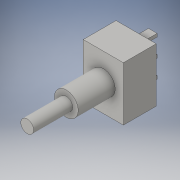
# Autodesk Inventor part: Mini toggle switch
Saved by Autodesk Inventor 2016 (Build 200138000, 138)
## iProperties
Created: 2017-09-11
Part Number: Mini toggle switch
Material: Generic
Document SubType Name: Modeling
Designer: student
Density: 1 g/cm^3
Appearance: Default
Author: student
Autodesk Inventor part; units mm, degrees
ref_plane "YZ Plane" through (0, 0, 0) normal (1, 0, 0) x (0, 1, 0)
ref_plane "XZ Plane" through (0, 0, 0) normal (0, 1, 0) x (-1, 0, 0)
ref_plane "XY Plane" through (0, 0, 0) normal (0, 0, 1) x (1, 0, 0)
sketch "Sketch1" plane through (0, 0, 0) normal (0, 0, 1) x (1, 0, 0)
  line L0 (-4.8133, 6.477) -> (4.8133, 6.477)
  line L1 (4.8133, 6.477) -> (4.8133, -6.477)
  line L2 (4.8133, -6.477) -> (-4.8133, -6.477)
  line L3 (-4.8133, -6.477) -> (-4.8133, 6.477)
  line L4 (-4.8133, 6.477) -> (4.8133, -6.477) construction
  line L5 (4.8133, 6.477) -> (-4.8133, -6.477) construction
  point P0 (0, 0)
  constraints: 12 end point, 2 midpoint, 2 parallel, 1 horizontal, 1 perpendicular
extrude "Extrusion1" add sketch "Sketch1" along normal blind 7.874
sketch "Sketch2" plane through (0, 0, 0) normal (0, 0, -1) x (-1, 0, 0)
  line L0 (-1.0414, 4.7498) -> (1.0414, 4.7498)
  line L1 (1.0414, 4.7498) -> (1.0414, 3.9878)
  line L2 (1.0414, 3.9878) -> (-1.0414, 3.9878)
  line L3 (-1.0414, 3.9878) -> (-1.0414, 4.7498)
  line L4 (-1.0414, 4.7498) -> (1.0414, 3.9878) construction
  line L5 (1.0414, 4.7498) -> (-1.0414, 3.9878) construction
  line L6 (4.8133, 6.477) -> (-4.8133, 6.477) projected
  point P0 (0, 0)
  point P1 (0, 4.3688)
  dimension "d7" = 2.0828
  dimension "d8" = 0.762
  dimension "d28" = 1.7272
  constraints: 12 end point, 2 midpoint, 2 parallel, 1 horizontal, 1 perpendicular
  measures "d7" distance of L1.end L2.end
  measures "d8" distance of L1.end L0.end
  measures "d28" distance between parallel lines of L6 L0
extrude "Extrusion2" add sketch "Sketch2" along normal blind 3.9878
sketch "Sketch3" plane through (0, 0, 0) normal (0, 0, -1) x (-1, 0, 0)
  line L0 (-1.0414, 0.381) -> (1.0414, 0.381)
  line L1 (1.0414, 0.381) -> (1.0414, -0.381)
  line L2 (1.0414, -0.381) -> (-1.0414, -0.381)
  line L3 (-1.0414, -0.381) -> (-1.0414, 0.381)
  line L4 (-1.0414, 0.381) -> (1.0414, -0.381) construction
  line L5 (1.0414, 0.381) -> (-1.0414, -0.381) construction
  line L6 (-1.0414, 3.9878) -> (1.0414, 3.9878) projected
  line L7 (4.8133, 6.477) -> (-4.8133, 6.477) projected
  line L8 (1.0414, 4.7498) -> (-1.0414, 4.7498) projected
  point P0 (0, 0)
  point P1 (0, 0)
  dimension "d13" = 2.0828
  dimension "d15" = 0.762
  dimension "d16" = 3.6068
  dimension "d18" = 1.7272
  constraints: 12 end point, 2 midpoint, 2 parallel, 1 horizontal, 1 perpendicular
  measures "d13" distance of L1.end L2.end
  measures "d15" distance of L1.end L0.end
  measures "d16" distance between parallel lines of L0 L6
  measures "d18" distance between parallel lines of L7 L8
extrude "Extrusion3" add sketch "Sketch3" along normal blind 3.9878
sketch "Sketch4" plane through (0, 0, 0) normal (0, 0, -1) x (-1, 0, 0)
  line L0 (-1.0414, -3.9878) -> (1.0414, -3.9878)
  line L1 (1.0414, -3.9878) -> (1.0414, -4.7498)
  line L2 (1.0414, -4.7498) -> (-1.0414, -4.7498)
  line L3 (-1.0414, -4.7498) -> (-1.0414, -3.9878)
  line L4 (-1.0414, -3.9878) -> (1.0414, -4.7498) construction
  line L5 (1.0414, -3.9878) -> (-1.0414, -4.7498) construction
  line L6 (-1.0414, -0.381) -> (1.0414, -0.381) projected
  line L7 (-4.8133, -6.477) -> (4.8133, -6.477) projected
  point P0 (0, 0)
  point P1 (0, -4.3688)
  dimension "d24" = 0.762
  dimension "d25" = 3.6068
  dimension "d27" = 2.0828
  constraints: 12 end point, 2 midpoint, 2 parallel, 1 horizontal, 1 perpendicular
  measures "d24" distance of L1.end L0.end
  measures "d25" distance between parallel lines of L6 L0
  measures "d27" distance of L1.end L2.end
extrude "Extrusion4" add sketch "Sketch4" along normal blind 3.9878
sketch "Sketch5" plane through (0, 0, 7.874) normal (0, 0, 1) x (1, 0, 0)
  circle A0 centre (0, 0) radius 2.8448
  dimension "d31" = 5.6896
  constraints: 2 coincident, 1 centre point
  measures "d31" diameter of A0
extrude "Extrusion5" add sketch "Sketch5" along normal blind 8.8646
sketch "Sketch6" plane through (0, 0, 16.7386) normal (0, 0, 1) x (1, 0, 0)
  circle A0 centre (0, 0) radius 1.5367
  dimension "d34" = 3.0734
  constraints: 1 centre point, 1 coincident
  measures "d34" diameter of A0
extrude "Extrusion6" add sketch "Sketch6" along normal blind 9.3726
body "Solid1"
